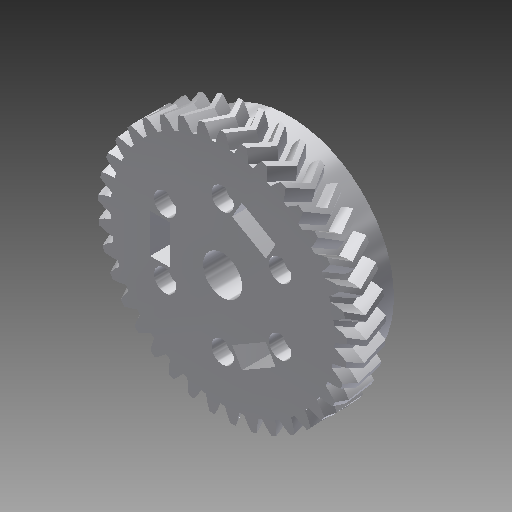
# Autodesk Inventor part: Spur Gear1
Saved by Autodesk Inventor 2017 SP1 (Build 210196100, 196)
## iProperties
Created: 2017-10-23
Part Number: Spur Gear1
Material: ABS Plastic
Document SubType Name: Modeling
Designer: Zach
Categories: <?xml version="1.0" encoding="UTF-16"?> <MemberInstance><Categories><FamilyTemplate><FamilyTemplateParameter ValueType="xs:double" Id="1" ObjectReferenceKey="da_z" ObjectType="kUserParameterObject"/><FamilyTemplateParameter ValueType="xs:double" Id="2" ObjectReferenceKey="da_b" ObjectType="kUserParameterObject"/><FamilyTemplateParameter ValueType="xs:double" Id="3" ObjectReferenceKey="da_beta" ObjectType="kUserParameterObject"/><FamilyTemplateParameter ValueType="xs:double" Id="4" ObjectReferenceKey="da_da" ObjectType="kUserParameterObject"/><FamilyTemplateParameter ValueType="xs:double" Id="5" ObjectReferenceKey="da_aw" ObjectType="kUserParameterObject"/><FamilyTemplateParameter ValueType="xs:string" Id="6" ObjectReferenceKey="EAIAABAAAACIAQAAAAAAAIAAAAAAAAAA" ObjectType="83910656" SubObjectId="SurfaceGeometry"/></FamilyTemplate><ParamToTemplateMap><ParamToTemplate CategoryParameter="//CategoryParameter[@InternalName='046C89C9-8512-4d59-83FE-43B91F4F132A']" TemplateParameter="1"/><ParamToTemplate CategoryParameter="//CategoryParameter[@InternalName='2552DF32-E462-4b46-AEBF-C6C7768E72AC']" TemplateParameter="2"/><ParamToTemplate CategoryParameter="//CategoryParameter[@InternalName='C9EE641D-15FC-4fae-A226-E94C4372FDD7']" TemplateParameter="3"/><ParamToTemplate><ParamToTemplate CategoryParameter="//CategoryParameter[@InternalName='00B6519A-459B-49c7-AD84-2E56D39A5744']" ConstantValue="0.000000"/></ParamToTemplate><ParamToTemplate><ParamToTemplate CategoryParameter="//CategoryParameter[@InternalName='04B31F0E-C7A6-4894-AA32-9629BEFACF47']" ConstantValue="1.000000"/></ParamToTemplate><ParamToTemplate><ParamToTemplate CategoryParameter="//CategoryParameter[@InternalName='43CBEC2E-7847-49e7-A936-2F7889FCB2D9']" ConstantValue="0.250000"/></ParamToTemplate><ParamToTemplate><ParamToTemplate CategoryParameter="//CategoryParameter[@InternalName='B1EFC894-105D-4ebd-86BF-FA20ED196853']" ConstantValue="0.350000"/></ParamToTemplate><ParamToTemplate><ParamToTemplate CategoryParameter="//CategoryParameter[@InternalName='51175063-3D10-4879-93E8-6246FE8B403D']" ConstantValue="2060000000.000000"/></ParamToTemplate><ParamToTemplate><ParamToTemplate CategoryParameter="//CategoryParameter[@InternalName='A3A52E27-4454-46a9-B0BD-C932399B70AF']" ConstantValue="0.300000"/></ParamToTemplate><ParamToTemplate><ParamToTemplate CategoryParameter="//CategoryParameter[@InternalName='91B76062-C214-41d9-B1B9-14D2AB99603D']" ConstantValue="0.200000"/></ParamToTemplate><ParamToTemplate><ParamToTemplate CategoryParameter="//CategoryParameter[@InternalName='374E806E-8B8A-4dda-A9AA-1039D6500AD2']" ConstantValue="5.000000"/></ParamToTemplate><ParamToTemplate><ParamToTemplate CategoryParameter="//CategoryParameter[@InternalName='2D373A89-B862-43d6-8D0B-0CBF12AB9F6C']" ConstantValue="0.392699"/></ParamToTemplate><ParamToTemplate CategoryParameter="//CategoryParameter[@InternalName='37777632-D6A2-4fac-9D53-DB8ACD95C989']" TemplateParameter="4"/><ParamToTemplate CategoryParameter="//CategoryParameter[@InternalName='FD1017F1-B727-4f7e-9707-0F86F1FF9423']" TemplateParameter="5"/><ParamToTemplate><ParamToTemplate CategoryParameter="//CategoryParameter[@InternalName='9E1B4470-B2D3-4ff1-B813-535BB4CDF51A']" ConstantValue="3520000.000000"/></ParamToTemplate><ParamToTemplate><ParamToTemplate CategoryParameter="//CategoryParameter[@InternalName='F8452263-BFF6-458c-9FB1-07C4B99E95CD']" ConstantValue="11400000.000000"/></ParamToTemplate><ParamToTemplate><ParamToTemplate CategoryParameter="//CategoryParameter[@InternalName='3E3BB259-FD49-497f-8171-6EBC954A3479']" ConstantValue="2.000000"/></ParamToTemplate><ParamToTemplate CategoryParameter="//CategoryParameter[@InternalName='27C3BAF2-7550-4e4b-AE2C-0DB134B7D9B7']" TemplateParameter="6"/></ParamToTemplateMap><Category DisplayName="Gear" InternalName="DC85795E-93AB-48d5-8EEE-5A27447B64BD" Mnemonic="Gear"><CategoryParameter DisplayName="z" InternalName="046C89C9-8512-4d59-83FE-43B91F4F132A" Mnemonic="z"/><CategoryParameter DisplayName="b" InternalName="2552DF32-E462-4b46-AEBF-C6C7768E72AC" Mnemonic="b"/><CategoryParameter DisplayName="||b|" InternalName="C9EE641D-15FC-4fae-A226-E94C4372FDD7" Mnemonic="beta"/><CategoryParameter DisplayName="x" InternalName="00B6519A-459B-49c7-AD84-2E56D39A5744" Mnemonic="x"/><CategoryParameter DisplayName="a*" InternalName="04B31F0E-C7A6-4894-AA32-9629BEFACF47" Mnemonic="a"/><CategoryParameter DisplayName="c*" InternalName="43CBEC2E-7847-49e7-A936-2F7889FCB2D9" Mnemonic="c"/><CategoryParameter DisplayName="r|.f|*" InternalName="B1EFC894-105D-4ebd-86BF-FA20ED196853" Mnemonic="rf"/><CategoryParameter DisplayName="E" InternalName="51175063-3D10-4879-93E8-6246FE8B403D" Mnemonic="E"/><CategoryParameter DisplayName="||m|" InternalName="A3A52E27-4454-46a9-B0BD-C932399B70AF" Mnemonic="mi"/><Category DisplayName="SpurGear" InternalName="26C5A22E-A91E-4dfd-A3B3-23CCAFAE1764" Mnemonic="SpurGear"><CategoryParameter DisplayName="m" InternalName="91B76062-C214-41d9-B1B9-14D2AB99603D" Mnemonic="m"/><CategoryParameter DisplayName="P" InternalName="374E806E-8B8A-4dda-A9AA-1039D6500AD2" Mnemonic="PP"/><CategoryParameter DisplayName="||a|" InternalName="2D373A89-B862-43d6-8D0B-0CBF12AB9F6C" Mnemonic="alpha"/><CategoryParameter DisplayName="d|.a|" InternalName="37777632-D6A2-4fac-9D53-DB8ACD95C989" Mnemonic="da"/><CategoryParameter DisplayName="a|.w|" InternalName="FD1017F1-B727-4f7e-9707-0F86F1FF9423" Mnemonic="aw"/><CategoryParameter DisplayName="||s||.Flim|" InternalName="9E1B4470-B2D3-4ff1-B813-535BB4CDF51A" Mnemonic="sFlim"/><CategoryParameter DisplayName="||s||.Hlim|" InternalName="F8452263-BFF6-458c-9FB1-07C4B99E95CD" Mnemonic="sHlim"/><CategoryParameter DisplayName="type" InternalName="3E3BB259-FD49-497f-8171-6EBC954A3479" Mnemonic="type"/><CategoryParameter DisplayName="PitchDiameter" InternalName="27C3BAF2-7550-4e4b-AE2C-0DB134B7D9B7" Mnemonic="IDS_PITCHDIAM"/></Category></Category></Categories></MemberInstance>
Density: 1.06 g/cm^3
Appearance: CR White
CustomPartVersion: 1
Author: Zach
Autodesk Inventor part; units mm, degrees
sketch "Sketch1" plane through (0, 0, 0) normal (0, 0, 1) x (1, 0, 0)
  circle A0 centre (0, 0) radius 44.7201
  dimension "d0" = 89.4403
  constraints: 1 centre point
  measures "d0" diameter of A0
extrude "Extrusion1" add sketch "Sketch1" along normal blind 7
ref_plane "Work Plane2" through (0, 0, 3.5) normal (0, 0, 1) x (1, 0, 0)
sketch "Sketch2" plane through (0, 0, 0) normal (0, 0, -1) x (-1, 0, 0)
  circle A0 centre (0, 0) radius 44.7201 projected
  circle A1 centre (0, 0) radius 42.9464
  dimension "d3" = 85.8929
  constraints: 1 centre point, 1 coincident
  measures "d3" diameter of A1
surface extrude "Pitch Diameter" sketch "Sketch2" against normal through all shown no curves A1
ref_plane "Work Plane8" through (0, 0, 0) normal (0.9963975, 0.0848059, 0) x (0, 0, 1)
ref_plane "Work Plane9" through (0, 0, 0) normal (1, 0, 0) x (0, 1, 0)
spur gear teeth "Spur Gear" teeth 37 pitch diameter 85.4478 tip diameter 89.4403 root diameter 80.4478 face width 7 helix angle 30 hand left start plane through (0, 0, 0) normal (0, 0, -1) x (-1, 0, 0)
mirror "Mirror1" about plane through (0, 0, 7) normal (0, 0, 1)
sketch "Sketch3" plane through (0, 0, 0) normal (0, 0, -1) x (-1, 0, 0)
  circle A0 centre (0, 0) radius 7
  circle A1 centre (0, -23.8125) radius 2.5
  circle A2 centre (20.6222, -11.9063) radius 2.5
  circle A3 centre (20.6222, 11.9062) radius 2.5
  circle A4 centre (0, 23.8125) radius 2.5
  circle A5 centre (-20.6222, 11.9063) radius 2.5
  circle A6 centre (-20.6222, -11.9062) radius 2.5
  line L0 (26, 7) -> (19, 7)
  line L1 (19, 7) -> (19, -7)
  line L2 (19, -7) -> (26, -7)
  line L3 (26, -7) -> (26, 7)
  line L4 (-19.0622, 19.0167) -> (-15.5622, 12.9545)
  line L5 (-15.5622, 12.9545) -> (-3.4378, 19.9545)
  line L6 (-3.4378, 19.9545) -> (-6.9378, 26.0167)
  line L7 (-6.9378, 26.0167) -> (-19.0622, 19.0167)
  line L8 (-6.9378, -26.0167) -> (-3.4378, -19.9545)
  line L9 (-3.4378, -19.9545) -> (-15.5622, -12.9545)
  line L10 (-15.5622, -12.9545) -> (-19.0622, -19.0167)
  line L11 (-19.0622, -19.0167) -> (-6.9378, -26.0167)
  point P0 (19, 0)
  point P1 (-9.5, 16.4545)
  point P2 (-9.5, -16.4545)
  dimension "d49" = 14
  dimension "d50" = 5
  dimension "d51" = 23.8125
  dimension "d54" = 360
  dimension "d56" = 7
  dimension "d57" = 14
  dimension "d58" = 19
  dimension "d61" = 360
  constraints: 24 end point, 7 centre point, 2 parallel, 1 coincident, 1 horizontal, 1 horizontal alignment, 1 midpoint, 1 perpendicular, 1 vertical alignment, 41 other
  measures "d49" diameter of A0
  measures "d50" diameter of A1
  measures "d51" distance of A1.centre point (0, 0)
  measures "d56" distance of L2.end L1.end
  measures "d57" distance of L1.end L0.end
  measures "d58" distance from line of point (0, 0) L1
extrude "Extrusion2" cut sketch "Sketch3" against normal through all
sketch "Sketch4" plane through (0, 0, 0) normal (0, 0, -1) x (-1, 0, 0)
  circle A0 centre (0, 0) radius 37.5
  line L0 (-15.5622, -12.9545) -> (-3.4378, -19.9545) projected
  line L1 (-3.4378, -19.9545) -> (-6.9378, -26.0167) projected
  line L2 (-6.9378, -26.0167) -> (-19.0622, -19.0167) projected
  line L3 (-19.0622, -19.0167) -> (-15.5622, -12.9545) projected
  line L4 (19, -7) -> (19, 7) projected
  line L5 (19, 7) -> (26, 7) projected
  line L6 (26, 7) -> (26, -7) projected
  line L7 (26, -7) -> (19, -7) projected
  circle A1 centre (-20.6222, 11.9063) radius 2.5 projected
  circle A2 centre (20.6222, 11.9062) radius 2.5 projected
  circle A3 centre (0, -23.8125) radius 2.5 projected
  circle A4 centre (20.6222, -11.9063) radius 2.5 projected
  circle A5 centre (0, 23.8125) radius 2.5 projected
  circle A6 centre (-20.6222, -11.9062) radius 2.5 projected
  line L8 (-3.4378, 19.9545) -> (-15.5622, 12.9545) projected
  line L9 (-15.5622, 12.9545) -> (-19.0622, 19.0167) projected
  line L10 (-19.0622, 19.0167) -> (-6.9378, 26.0167) projected
  line L11 (-6.9378, 26.0167) -> (-3.4378, 19.9545) projected
  circle A7 centre (0, 0) radius 7 projected
  arc A8 (0.9492, 44.7101) -> (-0.9492, 44.7101) centre (0, 0) ccw projected
  arc A9 (-6.6205, 44.2274) -> (-8.4916, 43.9065) centre (0, 0) ccw projected
  arc A10 (-13.9997, 42.4723) -> (-15.7897, 41.8399) centre (0, 0) ccw projected
  arc A11 (-20.9762, 39.4954) -> (-22.6335, 38.5696) centre (0, 0) ccw projected
  arc A12 (-27.3492, 35.3823) -> (-28.8263, 34.1897) centre (0, 0) ccw projected
  arc A13 (-32.9355, 30.2513) -> (-34.1897, 28.8263) centre (0, 0) ccw projected
  arc A14 (-37.5742, 24.2501) -> (-38.5696, 22.6335) centre (0, 0) ccw projected
  arc A15 (-41.1321, 17.5512) -> (-41.8399, 15.7897) centre (0, 0) ccw projected
  arc A16 (-43.5066, 10.3474) -> (-43.9065, 8.4916) centre (0, 0) ccw projected
  arc A17 (-44.6295, 2.8459) -> (-44.7101, 0.9492) centre (0, 0) ccw projected
  arc A18 (-44.4685, -4.7375) -> (-44.2274, -6.6205) centre (0, 0) ccw projected
  arc A19 (-43.0282, -12.1845) -> (-42.4723, -13.9997) centre (0, 0) ccw projected
  arc A20 (-40.3501, -19.2811) -> (-39.4954, -20.9762) centre (0, 0) ccw projected
  arc A21 (-36.5112, -25.8229) -> (-35.3823, -27.3492) centre (0, 0) ccw projected
  arc A22 (-31.6219, -31.6219) -> (-30.2513, -32.9355) centre (0, 0) ccw projected
  arc A23 (-25.8229, -36.5112) -> (-24.2501, -37.5742) centre (0, 0) ccw projected
  arc A24 (-19.2811, -40.3501) -> (-17.5512, -41.1321) centre (0, 0) ccw projected
  arc A25 (-12.1845, -43.0282) -> (-10.3474, -43.5066) centre (0, 0) ccw projected
  arc A26 (-4.7375, -44.4685) -> (-2.8459, -44.6295) centre (0, 0) ccw projected
  arc A27 (2.8459, -44.6295) -> (4.7375, -44.4685) centre (0, 0) ccw projected
  arc A28 (10.3474, -43.5066) -> (12.1845, -43.0282) centre (0, 0) ccw projected
  arc A29 (17.5512, -41.1321) -> (19.2811, -40.3501) centre (0, 0) ccw projected
  arc A30 (24.2501, -37.5742) -> (25.8229, -36.5112) centre (0, 0) ccw projected
  arc A31 (30.2513, -32.9355) -> (31.6219, -31.6219) centre (0, 0) ccw projected
  arc A32 (35.3823, -27.3492) -> (36.5112, -25.8229) centre (0, 0) ccw projected
  arc A33 (39.4954, -20.9762) -> (40.3501, -19.2811) centre (0, 0) ccw projected
  arc A34 (42.4723, -13.9997) -> (43.0282, -12.1845) centre (0, 0) ccw projected
  arc A35 (44.2274, -6.6205) -> (44.4685, -4.7375) centre (0, 0) ccw projected
  arc A36 (44.7101, 0.9492) -> (44.6295, 2.8459) centre (0, 0) ccw projected
  arc A37 (43.9065, 8.4916) -> (43.5066, 10.3474) centre (0, 0) ccw projected
  arc A38 (41.8399, 15.7897) -> (41.1321, 17.5512) centre (0, 0) ccw projected
  arc A39 (38.5696, 22.6335) -> (37.5742, 24.2501) centre (0, 0) ccw projected
  arc A40 (34.1897, 28.8263) -> (32.9355, 30.2513) centre (0, 0) ccw projected
  arc A41 (28.8263, 34.1897) -> (27.3492, 35.3823) centre (0, 0) ccw projected
  arc A42 (22.6335, 38.5696) -> (20.9762, 39.4954) centre (0, 0) ccw projected
  arc A43 (15.7897, 41.8399) -> (13.9997, 42.4723) centre (0, 0) ccw projected
  arc A44 (8.4916, 43.9065) -> (6.6205, 44.2274) centre (0, 0) ccw projected
  dimension "d65" = 75
  constraints: 1 centre point, 1 coincident, 1 horizontal alignment, 110 other
  measures "d65" diameter of A0
extrude "Extrusion3" add sketch "Sketch4" along normal blind 10
sketch "Sketch5" plane through (0, 0, 14) normal (0, 0, 1) x (0.985996, 0.1667687, 0)
  circle A0 centre (18.3478, -15.1787) radius 2.5 projected
  circle A1 centre (18.3478, -15.1787) radius 2.5 projected
  circle A2 centre (18.3478, -15.1787) radius 4
  circle A3 centre (22.319, 8.3004) radius 4
  circle A4 centre (3.9712, 23.479) radius 4
  circle A5 centre (-18.3478, 15.1787) radius 4
  circle A6 centre (-22.319, -8.3004) radius 4
  circle A7 centre (-3.9712, -23.479) radius 4
  point P0 (0, 0)
  dimension "d68" = 8
  dimension "d71" = 360
  constraints: 6 centre point, 1 coincident, 13 other
  measures "d68" diameter of A2
extrude "Extrusion4" cut sketch "Sketch5" against normal blind 5 contours A0 | A2 | A3 | A4 | A5 | A6 | A7
equation "\"d0\" = da_da"
equation "\"d1\" = da_b"
equation "\"d3\" = da_dw"
equation "\"d16\" = da_aw"
equation "\"d43\" = da_aw"
equation "\"d46\" = da_aw"
equation "\"da_da\" = 89.440269"
equation "\"da_b\" = 7"
equation "\"da_dw\" = 85.892857"
equation "\"da_aw\" = 65"
body "Solid1"
body "Srf1"
